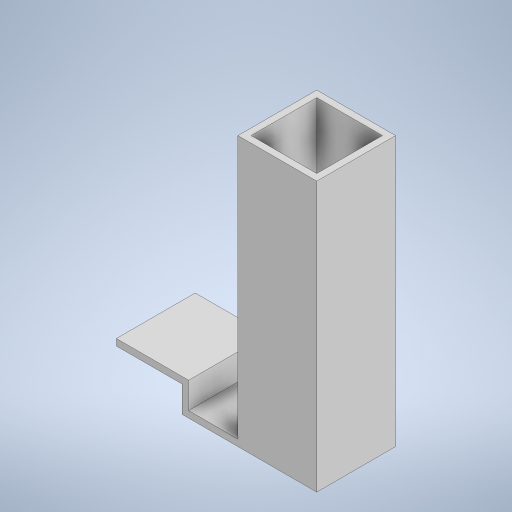
# Autodesk Inventor part: flexibler_standfuß_v0.3
Saved by Autodesk Inventor 2024 (Build 280153000, 153)
## iProperties
Created: 2023-10-27
Part Number: flexibler_standfuß_v0.3
Material: Generisch
Document SubType Name: Modeling
Designer: piuss
Density: 1 g/cm^3
Appearance: Vorgabe
Author: piuss
Autodesk Inventor part; units mm, degrees
ref_plane "YZ Plane" through (0, 0, 0) normal (1, 0, 0) x (0, 1, 0)
ref_plane "XZ Plane" through (0, 0, 0) normal (0, 1, 0) x (-1, 0, 0)
ref_plane "XY Plane" through (0, 0, 0) normal (0, 0, 1) x (1, 0, 0)
sketch "Skizze4" plane through (0, 0, 0) normal (0, 0, 1) x (1, 0, 0)
  line L0 (0, 0) -> (0, 2)
  line L1 (0, 2) -> (22, 2)
  line L2 (22, 2) -> (22, -6)
  line L3 (22, -6) -> (37, -6)
  line L4 (37, -6) -> (37, 74)
  line L5 (37, 74) -> (61, 74)
  line L6 (61, 74) -> (61, -8)
  line L7 (61, 74) -> (143, 74) construction
  line L8 (61, -8) -> (20, -8)
  line L9 (20, -8) -> (20, 0)
  line L10 (20, 0) -> (0, 0)
  dimension "d2" = 2
  dimension "d3" = 22
  dimension "d4" = 8
  dimension "d5" = 15
  dimension "d6" = 80
  dimension "d7" = 24
  dimension "d8" = 82
  dimension "d9" = 90
  dimension "d10" = 41
  constraints: 22 end point, 7 perpendicular, 2 parallel, 2 vertical, 1 horizontal
  measures "d2" distance of L0.start L0.end
  measures "d3" distance of L0.end L1.end
  measures "d4" distance of L1.end L2.end
  measures "d5" distance of L2.end L3.end
  measures "d6" distance of L3.end L4.end
  measures "d7" distance of L4.end L5.end
  measures "d8" distance of L5.end L6.end
  measures "d9" angle of L6 L7
  measures "d10" distance of L6.end L8.end
extrude "Extrusion3" add sketch "Skizze4" against normal blind 24
sketch "Skizze8" plane through (37, 74, 0) normal (0, 1, 0) x (1, 0, 0)
  line L0 (2, 2) -> (22, 2)
  line L1 (22, 2) -> (22, 22)
  line L2 (22, 22) -> (2, 22)
  line L3 (2, 22) -> (2, 2)
  point P0 (-37, 0)
  dimension "d23" = 20
  dimension "d24" = 20
  constraints: 8 end point, 2 parallel, 1 horizontal, 1 perpendicular
  measures "d23" distance of L2.end L1.end
  measures "d24" distance of L1.end L0.end
extrude "Extrusion5" cut sketch "Skizze8" against normal blind 200
